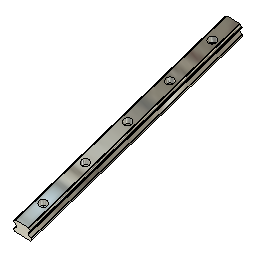
Parametric HGR20R Hiwin Rail v4 (Autodesk Fusion 360 design; units mm, degrees)
Autodesk Fusion 360 part; units mm, degrees
sketch "Sketch2" plane through (0, 0, 0) normal (0, 1, 0) x (1, 0, 0)
  line L0 (-504.5454, -6.5205) -> (-504.7356, -6.3303)
  arc A0 (-504.882, -5.9768) -> (-504.7356, -6.3303) centre (-504.382, -5.9768) ccw
  line L1 (-504.882, -5.9768) -> (-504.882, -4.9195)
  arc A1 (-504.7356, -4.566) -> (-504.882, -4.9195) centre (-504.382, -4.9195) ccw
  line L2 (-504.7356, -4.566) -> (-504.5574, -4.3878)
  arc A2 (-504.2944, -4.2496) -> (-504.5574, -4.3878) centre (-504.2038, -4.7413) ccw
  arc A3 (-504.2944, -4.2496) -> (-502.6657, -2.6209) centre (-504.6621, -2.2532) ccw
  arc A4 (-502.5275, -2.3579) -> (-502.6657, -2.6209) centre (-502.1739, -2.7114) ccw
  line L3 (-502.5275, -2.3579) -> (-501.7749, -1.6053)
  arc A5 (-501.7749, -1.6053) -> (-501.482, -0.8982) centre (-502.482, -0.8982) ccw
  line L4 (-501.482, -0.8982) -> (-501.482, 0.6619)
  arc A6 (-501.482, 0.6619) -> (-501.7749, 1.369) centre (-502.482, 0.6619) ccw
  line L5 (-501.7749, 1.369) -> (-504.5891, 4.1832)
  arc A7 (-504.882, 4.8903) -> (-504.5891, 4.1832) centre (-503.882, 4.8903) ccw
  line L6 (-504.882, 4.8903) -> (-504.882, 7.5468)
  line L7 (-504.882, 7.5468) -> (-503.882, 8.5468)
  line L8 (-503.882, 8.5468) -> (-485.882, 8.5468)
  line L9 (-485.882, 8.5468) -> (-484.882, 7.5468)
  line L10 (-484.882, 7.5468) -> (-484.882, 4.8903)
  arc A8 (-485.1749, 4.1832) -> (-484.882, 4.8903) centre (-485.882, 4.8903) ccw
  line L11 (-485.1749, 4.1832) -> (-487.9891, 1.369)
  arc A9 (-487.9891, 1.369) -> (-488.282, 0.6619) centre (-487.282, 0.6619) ccw
  line L12 (-488.282, 0.6619) -> (-488.282, -0.8982)
  arc A10 (-488.282, -0.8982) -> (-487.9891, -1.6053) centre (-487.282, -0.8982) ccw
  line L13 (-487.9891, -1.6053) -> (-487.2366, -2.3579)
  arc A11 (-487.0984, -2.6209) -> (-487.2366, -2.3579) centre (-487.5902, -2.7114) ccw
  arc A12 (-487.0984, -2.6209) -> (-485.4697, -4.2496) centre (-485.102, -2.2532) ccw
  arc A13 (-485.2067, -4.3878) -> (-485.4697, -4.2496) centre (-485.5603, -4.7413) ccw
  line L14 (-485.2067, -4.3878) -> (-485.0285, -4.566)
  arc A14 (-484.882, -4.9195) -> (-485.0285, -4.566) centre (-485.382, -4.9195) ccw
  line L15 (-484.882, -4.9195) -> (-484.882, -5.9768)
  arc A15 (-485.0285, -6.3303) -> (-484.882, -5.9768) centre (-485.382, -5.9768) ccw
  line L16 (-485.0285, -6.3303) -> (-485.2187, -6.5205)
  arc A16 (-485.4793, -6.6583) -> (-485.2187, -6.5205) centre (-485.5722, -6.167) ccw
  arc A17 (-485.4793, -6.6583) -> (-487.0966, -8.2756) centre (-485.102, -8.6529) ccw
  arc A18 (-487.2344, -8.5362) -> (-487.0966, -8.2756) centre (-487.5879, -8.1826) ccw
  line L17 (-487.2344, -8.5362) -> (-487.6513, -8.9532)
  line L18 (-487.6513, -8.9532) -> (-502.1128, -8.9532)
  line L19 (-502.1128, -8.9532) -> (-502.5297, -8.5362)
  arc A19 (-502.6674, -8.2756) -> (-502.5297, -8.5362) centre (-502.1762, -8.1826) ccw
  arc A20 (-502.6674, -8.2756) -> (-504.2848, -6.6583) centre (-504.6621, -8.6529) ccw
  arc A21 (-504.5454, -6.5205) -> (-504.2848, -6.6583) centre (-504.1918, -6.167) ccw
extrude "Extrude2" add sketch "Sketch2" along normal blind 300
hole "Hole2" at (-494.8818, 30, 8.9532) direction (0, 0, -1) diameter 6 depth 17.5 tip angle 118 counterbore diameter 9.5 counterbore depth 8.5
pattern_linear "R-Pattern2" count 5 spacing 60 along (0, 1, 0) of "Hole2"
equation "RailLength = 300 mm"
equation "RailHoleSpacing = 60 mm"
equation "RailNumberOfHoles = round(RailLength / RailHoleSpacing)"
equation "RailFirstHoleOffset = ( RailLength - ( ( RailNumberOfHoles - 1 ) * RailHoleSpacing ) ) / 2"
equation "d18 = RailLength"
equation "d25 = RailFirstHoleOffset"
equation "d27 = RailNumberOfHoles"
equation "d29 = RailHoleSpacing"
